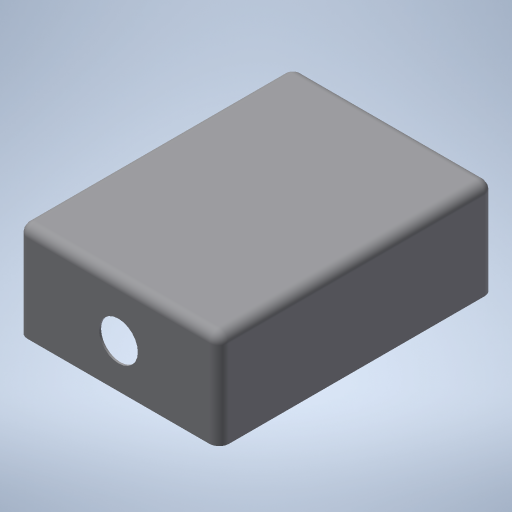
# Autodesk Inventor part: aja arduino 2
Saved by Autodesk Inventor 2023 (Build 270158000, 158)
## iProperties
Created: 2022-10-27
Part Number: aja arduino 2
Material: Generic
Document SubType Name: Modeling
Designer: Xiaba
Density: 1 g/cm^3
Appearance: Default
Author: Xiaba
Autodesk Inventor part; units mm, degrees
ref_plane "YZ Plane" through (0, 0, 0) normal (1, 0, 0) x (0, 1, 0)
ref_plane "XZ Plane" through (0, 0, 0) normal (0, 1, 0) x (-1, 0, 0)
ref_plane "XY Plane" through (0, 0, 0) normal (0, 0, 1) x (1, 0, 0)
sketch "Sketch1" plane through (0, 0, 0) normal (0, 1, 0) x (-1, 0, 0)
  line L0 (0, 0) -> (104, 0)
  line L1 (104, 0) -> (104, -142)
  line L2 (104, -142) -> (0, -142)
  line L3 (0, -142) -> (0, 0)
  dimension "d0" = 142
  dimension "d1" = 104
  constraints: 8 end point, 2 parallel, 1 horizontal, 1 perpendicular
  measures "d0" distance of L0.end L1.end
  measures "d1" distance of L1.end L2.end
extrude "Extrusion1" add sketch "Sketch1" along normal blind 50
fillet "Fillet1" radius 5 8 edges at (-104, 50, -71) (-52, 50, 0) (-52, 50, -142) (0, 50, -71) (0, 25, 0) (0, 25, -142) (-104, 25, 0) (-104, 25, -142)
shell "Shell1" thickness 1 removed faces 1 at (-34.6667, 0, -93)
sketch "Sketch2" plane through (-99, 0, 0) normal (0, 0, 1) x (1, 0, 0)
  line L0 (94, 45) -> (94, 0) projected
  line L1 (0, 45) -> (94, 45) projected
  line L2 (0, 0) -> (0, 45) projected
  line L3 (0, 0) -> (94, 0) projected
  circle A0 centre (47, 22.5) radius 10
  point P0 (99, 0)
  dimension "d6" = 20
  constraints: 1 centre point
  measures "d6" diameter of A0
extrude "Extrusion2" cut sketch "Sketch2" against normal blind 50 contours A0
sketch "Sketch3" plane through (-5, 0, -142) normal (0, 0, -1) x (-1, 0, 0)
  line L0 (0, 0) -> (0, 45) projected
  line L1 (0, 0) -> (94, 0) projected
  line L2 (94, 45) -> (94, 0) projected
  line L3 (0, 45) -> (94, 45) projected
  circle A0 centre (47, 22.5) radius 2.5
  point P0 (-5, 0)
  dimension "d9" = 5
  constraints: 1 centre point
  measures "d9" diameter of A0
extrude "Extrusion3" cut sketch "Sketch3" against normal blind 50 contours A0
body "Solid1"
